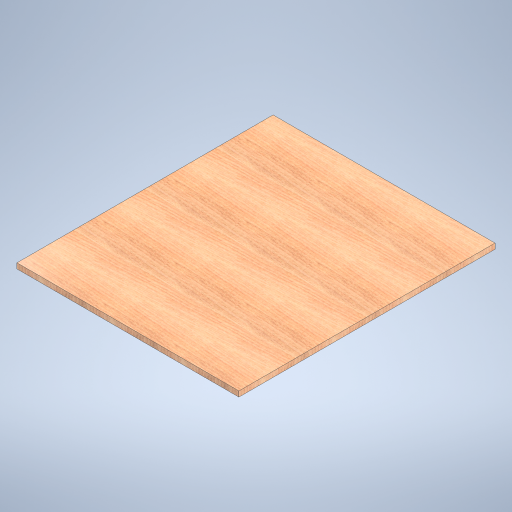
# Autodesk Inventor part: WoodBase
Saved by Autodesk Inventor 2024.2 (Build 282272000, 272)
## iProperties
Created: 2024-01-23
Part Number: WoodBase
Material: Wood (Birch)
Document SubType Name: Modeling
Designer: airso
Density: 0.55 g/cm^3
Appearance: Birch - Natural Polished
Author: airso
Autodesk Inventor part; units mm, degrees
ref_plane "YZ Plane" through (0, 0, 0) normal (1, 0, 0) x (0, 1, 0)
ref_plane "XZ Plane" through (0, 0, 0) normal (0, 1, 0) x (-1, 0, 0)
ref_plane "XY Plane" through (0, 0, 0) normal (0, 0, 1) x (1, 0, 0)
sketch "Sketch1" plane through (0, 0, 0) normal (0, 1, 0) x (-1, 0, 0)
  line L0 (-396.24, 457.2) -> (396.24, 457.2)
  line L1 (396.24, 457.2) -> (396.24, -457.2)
  line L2 (396.24, -457.2) -> (-396.24, -457.2)
  line L3 (-396.24, -457.2) -> (-396.24, 457.2)
  line L4 (-396.24, 457.2) -> (396.24, -457.2) construction
  line L5 (396.24, 457.2) -> (-396.24, -457.2) construction
  point P0 (0, 0)
  dimension "d0" = 914.4
  dimension "d1" = 792.48
  constraints: 12 end point, 2 midpoint, 2 parallel, 1 horizontal, 1 perpendicular
  measures "d0" distance of L0.end L1.end
  measures "d1" distance of L1.end L2.end
extrude "Extrusion1" add sketch "Sketch1" along normal blind 19.05
body "Solid1"
